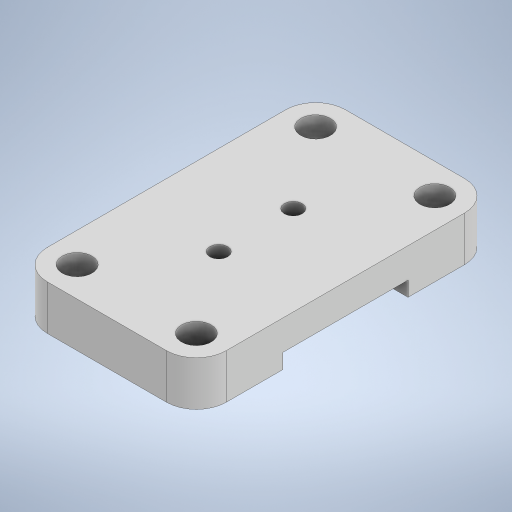
# Autodesk Inventor part: base_obj1
Saved by Autodesk Inventor 2023.2 (Build 272271030, 271C)
## iProperties
Created: 2023-02-25
Part Number: base_obj1
Material: Generic
Document SubType Name: Modeling
Designer: Cris Pat
Density: 1 g/cm^3
Appearance: Default
Author: Cris Pat
Autodesk Inventor part; units mm, degrees
ref_plane "YZ Plane" through (0, 0, 0) normal (1, 0, 0) x (0, 1, 0)
ref_plane "XZ Plane" through (0, 0, 0) normal (0, 1, 0) x (-1, 0, 0)
ref_plane "XY Plane" through (0, 0, 0) normal (0, 0, 1) x (1, 0, 0)
sketch "Sketch1" plane through (0, 0, 0) normal (0, 1, 0) x (-1, 0, 0)
  line L0 (30, 50) -> (-30, 50)
  line L1 (-30, 50) -> (-30, -50)
  line L2 (-30, -50) -> (30, -50)
  line L3 (30, -50) -> (30, 50)
  line L4 (30, 0) -> (-30, 0) construction
  line L5 (0, 50) -> (0, -50) construction
  circle A0 centre (20, 40) radius 5
  circle A1 centre (-20, 40) radius 5
  circle A2 centre (20, -40) radius 5
  circle A3 centre (-20, -40) radius 5
  circle A4 centre (0, -12.5) radius 3
  circle A5 centre (0, 12.5) radius 3
  point P0 (0, 0)
  point P1 (0, 0)
  dimension "d0" = 60
  dimension "d1" = 100
  dimension "d2" = 10
  dimension "d3" = 40
  dimension "d4" = 80
  dimension "d14" = 6
  dimension "d15" = 25
  constraints: 12 end point, 6 centre point, 4 midpoint, 4 symmetric about line, 2 parallel, 2 perpendicular, 1 coincident, 1 horizontal, 1 horizontal alignment, 1 point on line, 1 vertical alignment, 4 other
  measures "d0" distance of L2.end L1.end
  measures "d1" distance of L1.end L0.end
  measures "d2" diameter of A0
  measures "d3" distance of A1.centre A0.centre
  measures "d4" distance of A2.centre A0.centre
  measures "d14" diameter of A4
  measures "d15" distance of A5.centre A4.centre
extrude "Extrusion1" add sketch "Sketch1" along normal blind 15
fillet "Fillet1" radius 10 4 edges at (30, 7.5, 50) (30, 7.5, -50) (-30, 7.5, 50) (-30, 7.5, -50)
sketch "Sketch2" plane through (30, 0, 40) normal (1, 0, 0) x (0, 0, -1)
  line L0 (80, 15) -> (80, 0) construction
  line L1 (0, 15) -> (80, 15) construction
  line L2 (0, 0) -> (0, 15) construction
  line L3 (0, 0) -> (80, 0) construction
  line L4 (19, 5) -> (61, 5)
  line L5 (61, 5) -> (61, 0)
  line L6 (61, 0) -> (19, 0)
  line L7 (19, 0) -> (19, 5)
  line L8 (40, 0) -> (40, 15) construction
  line L9 (0, 15) -> (80, 15) construction
  point P0 (40, 5)
  dimension "d9" = 42
  dimension "d10" = 5
  constraints: 10 end point, 3 midpoint, 2 parallel, 1 horizontal, 1 horizontal alignment, 1 perpendicular, 1 vertical alignment
  measures "d9" distance of L5.end L6.end
  measures "d10" distance of L4.end L5.end
extrude "Extrusion2" cut sketch "Sketch2" against normal through all
body "Solid1"
